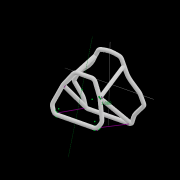
# Autodesk Inventor part: profiles
Saved by Autodesk Inventor 2020 (Build 240168000, 168)
## iProperties
Created: 2020-03-12
Part Number: profiles
Material: Generic
Document SubType Name: Modeling
Designer: valer
Density: 1 g/cm^3
Appearance: Default
Author: valer
Autodesk Inventor part; units mm, degrees
ref_plane "YZ Plane" through (0, 0, 0) normal (1, 0, 0) x (0, 1, 0)
ref_plane "XZ Plane" through (0, 0, 0) normal (0, 1, 0) x (-1, 0, 0)
sketch "FrontTube" plane through (0, 0, 0) normal (1, 0, 0) x (0, 1, 0)
  circle A0 centre (203.2, 0) radius 12.7
  line L0 (-302.2779, 0) -> (302.263, 0) projected
  point P0 (0, 0)
  dimension "d35" = 25.4
  constraints: 1 centre point, 1 point on line
  measures "d35" diameter of A0
sketch "Front1" plane through (0, 0, 0) normal (0, 0, 1) x (1, 0, 0)
  arc A0 (63.0606, 202.3316) -> (0.9117, 211.6354) centre (-9.1171, -67.5845) ccw
  arc A1 (86.36, 182.4422) -> (63.0606, 202.3316) centre (53.8743, 167.9787) ccw
  line L0 (0, 211.6667) -> (0, -211.6667) construction
  line L1 (86.36, 182.4422) -> (117.3533, 112.8301)
  line L2 (149.1123, 68.3056) -> (198.6494, 22.1116)
  line L3 (213.8608, 1.1748) -> (235.3298, -44.8656)
  line L4 (232.2048, -71.3906) -> (184.8333, -131.0763)
  line L5 (137.16, -211.6667) -> (0, -211.6667)
  line L6 (170.9584, -158.5658) -> (161.6802, -192.894)
  arc A2 (117.3533, 112.8301) -> (149.1123, 68.3056) centre (242.6552, 168.6181) ccw
  arc A3 (137.16, -211.6667) -> (161.6802, -192.894) centre (137.16, -186.2667) ccw
  arc A4 (184.8333, -131.0763) -> (170.9584, -158.5658) centre (244.5189, -178.4478) ccw
  arc A5 (232.2048, -71.3906) -> (235.3298, -44.8656) centre (212.3096, -55.6001) ccw
  arc A6 (213.8608, 1.1748) -> (198.6494, 22.1116) centre (152.4, -27.4848) ccw
  arc A7 (-0.9117, 211.6354) -> (-63.0606, 202.3316) centre (9.1171, -67.5845) ccw
  arc A8 (-63.0606, 202.3316) -> (-86.36, 182.4422) centre (-53.8743, 167.9787) ccw
  line L7 (-86.36, 182.4422) -> (-117.3533, 112.8301)
  line L8 (-149.1123, 68.3056) -> (-198.6494, 22.1116)
  line L9 (-213.8608, 1.1748) -> (-235.3298, -44.8656)
  line L10 (-232.2048, -71.3906) -> (-184.8333, -131.0763)
  line L11 (-137.16, -211.6667) -> (0, -211.6667)
  line L12 (-170.9584, -158.5658) -> (-161.6802, -192.894)
  arc A9 (-149.1123, 68.3056) -> (-117.3533, 112.8301) centre (-242.6552, 168.6181) ccw
  arc A10 (-161.6802, -192.894) -> (-137.16, -211.6667) centre (-137.16, -186.2667) ccw
  arc A11 (-170.9584, -158.5658) -> (-184.8333, -131.0763) centre (-244.5189, -178.4478) ccw
  arc A12 (-235.3298, -44.8656) -> (-232.2048, -71.3906) centre (-212.3096, -55.6001) ccw
  arc A13 (-198.6494, 22.1116) -> (-213.8608, 1.1748) centre (-152.4, -27.4848) ccw
  arc A14 (0.9117, 211.6354) -> (-0.9117, 211.6354) centre (0, 186.2518) ccw
  point P0 (0, 0)
  point P1 (0, 0)
  dimension "d15" = 86.36
  dimension "d16" = 25.4
  dimension "d17" = 25.4
  dimension "d18" = 76.2
  dimension "d19" = 25
  dimension "d20" = 47
  dimension "d21" = 24
  dimension "d22" = 137.16
  dimension "d23" = 279.4
  dimension "d24" = 35.56
  dimension "d25" = 76.2
  dimension "d26" = 137.16
  dimension "d27" = 67.7333
  dimension "d28" = 50.8
  dimension "d29" = 76.2
  dimension "d30" = 35.56
  dimension "d32" = 152.4
  dimension "d33" = 43.688
  dimension "d34" = 423.3333
  dimension "d38" = 25.4
  constraints: 32 point on circle, 26 end point, 19 symmetric about line, 15 centre point, 14 tangent, 1 midpoint, 1 perpendicular, 1 vertical, 7 other
  measures "d15" distance from line of L1.start L0
  measures "d16" radius of A3
  measures "d17" radius of A5
  measures "d18" radius of A4
  measures "d19" angle of L0 L3
  measures "d20" angle of L0 L2
  measures "d21" angle of L0 L1
  measures "d22" distance of L5.start L0.end
  measures "d23" radius of A0
  measures "d24" radius of A1
  measures "d25" distance of L1.start L1.end
  measures "d26" radius of A2
  measures "d27" distance of L2.start L2.end
  measures "d28" distance of L3.start L3.end
  measures "d29" distance of L4.start L4.end
  measures "d30" distance of L6.start L6.end
  measures "d32" distance from line of L0 A6.centre
  measures "d33" vertical distance of A1.centre L0.start
  measures "d34" distance of L0.end L0.start
  measures "d38" radius of A14
sweep "Front1Feature" add profiles "FrontTube" path "Front1" path curves A0 A1 L1 A2 L2 A6 L3 A5 L4 A4 L6 A3 L5 L11 A10 L12 A11 L10 A12 L9 A13 L8 A9 L7 A8 A7 A14
ref_plane "MiddlePlane" through (0, 0, 254) normal (0, 0, 1) x (1, 0, 0)
sketch "MiddleEdge" plane through (0, 0, 254) normal (0, 0, 1) x (1, 0, 0)
  line L0 (-31.1191, 127.0482) -> (68.8934, 127.0482)
  point P0 (0, 0)
  constraints: 2 end point, 1 horizontal
ref_plane "MiddleRotatedPlane" through (-31.1191, 127.0482, 254) normal (0, 0.309017, 0.9510565) x (1, 0, 0)
ref_plane "BackPlane" through (0, 0, 457.2) normal (0, 0, 1) x (1, 0, 0)
sketch "Middle" plane through (-31.1191, 127.0482, 254) normal (0, 0.309017, 0.9510565) x (1, 0, 0)
  line L0 (31.1191, 38.7554) -> (75.1914, 38.7554)
  line L1 (105.257, 22.1842) -> (149.4691, -47.8183)
  line L2 (180.8254, -206.284) -> (188.7793, -192.1968)
  line L3 (154.4333, -58.0694) -> (191.3548, -162.9001)
  line L4 (31.1191, -224.3603) -> (149.8603, -224.3603)
  line L5 (31.1191, 38.7554) -> (31.1191, -224.3603) construction
  arc A0 (105.257, 22.1842) -> (75.1914, 38.7554) centre (75.1914, 3.1954) ccw
  arc A1 (154.4333, -58.0694) -> (149.4691, -47.8183) centre (106.5183, -74.9451) ccw
  arc A2 (188.7793, -192.1968) -> (191.3548, -162.9001) centre (157.8143, -174.7131) ccw
  arc A3 (149.8603, -224.3603) -> (180.8254, -206.284) centre (149.8603, -188.8003) ccw
  line L6 (31.1191, 38.7554) -> (-12.9532, 38.7554)
  line L7 (-43.0188, 22.1842) -> (-87.2309, -47.8183)
  line L8 (-118.5871, -206.284) -> (-126.5411, -192.1968)
  line L9 (-92.1951, -58.0694) -> (-129.1166, -162.9001)
  line L10 (31.1191, -224.3603) -> (-87.6221, -224.3603)
  arc A4 (-12.9532, 38.7554) -> (-43.0188, 22.1842) centre (-12.9532, 3.1954) ccw
  arc A5 (-87.2309, -47.8183) -> (-92.1951, -58.0694) centre (-44.2801, -74.9451) ccw
  arc A6 (-129.1166, -162.9001) -> (-126.5411, -192.1968) centre (-95.5761, -174.7131) ccw
  arc A7 (-118.5871, -206.284) -> (-87.6221, -224.3603) centre (-87.6221, -188.8003) ccw
  line L11 (31.1191, 38.7554) -> (31.1191, 45.1054) construction
  line L12 (31.1191, -224.3603) -> (31.1191, -275.1603) construction
  point P0 (31.1191, -42.3397)
  dimension "d86" = 35.56
  dimension "d87" = 50.8
  dimension "d88" = 35.56
  dimension "d98" = 50.8
  constraints: 26 end point, 16 point on circle, 12 symmetric about line, 8 centre point, 8 tangent, 3 vertical, 2 horizontal, 1 equal radius, 4 other
  measures "d86" radius of A0
  measures "d87" radius of A1
  measures "d88" radius of A2
  measures "d98" distance of L4.start L12.end
sketch "MiddleTube" plane through (0, 0, 0) normal (1, 0, 0) x (0, 1, 0)
  circle A0 centre (163.9068, 242.0239) radius 12.7
  point P0 (0, 0)
  dimension "d89" = 25.4
  constraints: 1 centre point, 1 coincident
  measures "d89" diameter of A0
sweep "MiddleFeature" add profiles "MiddleTube" path "Middle" separate body path curves L6 A4 L7 A5 L9 A6 L8 A7 L10 L4 A3 L2 A2 L3 A1 L1 A0 L0
sketch "BackProfile" plane through (0, 0, 457.2) normal (0, 0, 1) x (1, 0, 0)
  line L0 (41.4631, 93.1618) -> (47.5828, 84.9091)
  line L1 (0, 100.0125) -> (27.8545, 100.0125)
  line L2 (50.6768, 77.6546) -> (60.2398, 21.3464)
  line L3 (0, 1.5679) -> (43.5372, 1.5679)
  line L4 (0, 100.0125) -> (0, 1.5679) construction
  arc A0 (41.4631, 93.1618) -> (27.8545, 100.0125) centre (27.8545, 83.0707) ccw
  arc A1 (50.6768, 77.6546) -> (47.5828, 84.9091) centre (33.9742, 74.8179) ccw
  arc A2 (43.5372, 1.5679) -> (60.2398, 21.3464) centre (43.5372, 18.5097) ccw
  line L5 (-41.4631, 93.1618) -> (-47.5828, 84.9091)
  line L6 (0, 100.0125) -> (-27.8545, 100.0125)
  line L7 (-50.6768, 77.6546) -> (-60.2398, 21.3464)
  line L8 (0, 1.5679) -> (-43.5372, 1.5679)
  arc A3 (-27.8545, 100.0125) -> (-41.4631, 93.1618) centre (-27.8545, 83.0707) ccw
  arc A4 (-47.5828, 84.9091) -> (-50.6768, 77.6546) centre (-33.9742, 74.8179) ccw
  arc A5 (-60.2398, 21.3464) -> (-43.5372, 1.5679) centre (-43.5372, 18.5097) ccw
  line L9 (0, 100.0125) -> (0, 125.3956) construction
  point P0 (0, 0)
  dimension "d92" = 16.9418
  dimension "d93" = 16.9418
  dimension "d97" = 25.3831
  constraints: 20 end point, 12 point on circle, 9 symmetric about line, 6 centre point, 6 tangent, 2 horizontal, 2 vertical, 1 equal radius, 3 other
  measures "d92" radius of A0
  measures "d93" radius of A2
  measures "d97" distance of L1.start L9.end
sketch "BackTube" plane through (0, 0, 0) normal (1, 0, 0) x (0, 1, 0)
  circle A0 centre (100.0125, 457.2) radius 12.7
  point P0 (0, 0)
  point P1 (100.0125, 457.2)
  point P2 (100.0125, 457.2)
  point P3 (100.0125, 457.2)
  dimension "d94" = 25.4
  constraints: 1 centre point, 1 coincident
  measures "d94" diameter of A0
feature "BackFeature" [suppressed]
sketch "FrontTopTubes" plane through (0, 0, 0) normal (0, 0, 1) x (1, 0, 0)
  circle A0 centre (94.1356, 144.1985) radius 12.7
  line L0 (57.5964, 181.8978) -> (64.158, 206.4357) projected
  line L1 (0.6083, 203.1891) -> (0.6083, 203.1891) projected
  line L2 (0.6083, 203.1891) -> (0.6083, 203.1891) projected
  line L3 (-0.1525, 190.4973) -> (-1.0642, 215.8809) projected
  line L4 (-57.5964, 181.8978) -> (-64.158, 206.4357) projected
  line L5 (-137.16, -190.5149) -> (-137.16, -215.9149) projected
  line L6 (137.16, -190.5149) -> (137.16, -215.9149) projected
  line L7 (98.0302, 104.2269) -> (121.2343, 114.558) construction
  line L8 (67.0369, 173.839) -> (90.2409, 184.1701) projected
  line L9 (90.2409, 184.1701) -> (121.2343, 114.558) construction
  line L10 (67.0369, 173.839) -> (98.0302, 104.2269) construction
  line L11 (67.0369, 173.839) -> (90.2409, 184.1701) projected
  line L12 (0, -302.274) -> (0, 302.2401) construction
  circle A1 centre (-94.1356, 144.1985) radius 12.7
  circle A2 centre (147.4628, -199.7238) radius 12.7
  circle A3 centre (-147.4628, -199.7238) radius 12.7
  arc A4 (-141.2611, -187.3751) -> (-137.16, -190.5149) centre (-137.16, -186.2667) ccw projected
  arc A5 (-165.7812, -194.0025) -> (-137.16, -215.9149) centre (-137.16, -186.2667) ccw projected
  arc A6 (137.16, -215.9149) -> (165.7812, -194.0025) centre (137.16, -186.2667) ccw projected
  point P0 (0, 0)
  point P1 (155.1831, -209.8078)
  point P2 (-155.1831, -209.8078)
  dimension "d99" = 25.4
  dimension "d100" = 38.1
  constraints: 2 centre point, 2 coincident, 2 point on circle, 1 symmetric about line, 1 tangent, 10 other
  measures "d99" diameter of A0
  measures "d100" distance from line of L8 A0.centre
sketch "MiddleTopTubes" plane through (-31.1191, 127.0482, 254) normal (0, 0.309017, 0.9510565) x (1, 0, 0)
  circle A0 centre (152.2394, -52.8043) radius 12.7
  line L0 (115.9947, 28.9659) -> (94.5193, 15.4025) construction
  line L1 (31.1191, -430.2644) -> (31.1191, 261.8485) construction
  circle A1 centre (-90.0012, -52.8043) radius 12.7
  arc A2 (142.4545, -62.2883) -> (138.7314, -54.6) centre (106.5183, -74.9451) ccw projected
  arc A3 (166.4121, -53.8505) -> (160.2068, -41.0366) centre (106.5183, -74.9451) ccw projected
  circle A4 centre (167.7879, -219.5105) radius 12.7
  circle A5 centre (-105.5496, -219.5105) radius 12.7
  arc A6 (149.8603, -237.0603) -> (191.8843, -212.5281) centre (149.8603, -188.8003) ccw projected
  arc A7 (149.8603, -211.6603) -> (169.7664, -200.0398) centre (149.8603, -188.8003) ccw projected
  arc A8 (-129.6461, -212.5281) -> (-87.6221, -237.0603) centre (-87.6221, -188.8003) ccw projected
  arc A9 (-107.5282, -200.0398) -> (-87.6221, -211.6603) centre (-87.6221, -188.8003) ccw projected
  point P0 (31.1191, -42.3397)
  point P1 (163.6697, -47.269)
  point P2 (174.1906, -230.4784)
  point P3 (-111.9523, -230.4784)
  dimension "d106" = 25.4
  constraints: 3 point on circle, 2 coincident, 1 centre point, 1 symmetric about line, 13 other
sketch3d "TopTubeLeft"
  line L0 (121.1203, 76.8284, 270.3174) -> (94.1356, 144.1985, 0)
sweep "TopTubeLeftFeature" add profiles "MiddleTopTubes" path "TopTubeLeft" separate body contours A0
sketch3d "TopTubeRight"
  line L0 (-94.1356, 144.1985, 0) -> (-121.1203, 76.8284, 270.3174)
sweep "TopTubeRightFeature" add profiles "FrontTopTubes" path "TopTubeRight" separate body contours A1
sketch3d "BottomTubeRight"
sketch3d "BottomTubeLeft"
ref_plane "SideTubeRightPlane" through (121.1203, 76.8284, 270.3174) normal (0.0679602, -0.7134686, -0.6973837) x (0.995494, 0.0948241, 0)
ref_plane "SideTubeLeftPlane" through (-121.1203, 76.8284, 270.3174) normal (0.0679602, 0.7134686, 0.6973837) x (-0.995494, 0.0948241, 0)
sketch "SideTubeRightProfile" plane through (121.1203, 76.8284, 270.3174) normal (0.0679602, -0.7134686, -0.6973837) x (0.995494, 0.0948241, 0)
  circle A0 centre (0, 0) radius 12.7
  ellipse E0 centre (0, 0) end of major axis (12.6751, -0.7952) minor radius 11.2233 projected
  point P0 (-127.8597, -148.408)
  dimension "d113" = 25.4
  constraints: 1 centre point, 1 coincident
  measures "d113" diameter of A0
sketch "SideTubeLeftProfile" plane through (-121.1203, 76.8284, 270.3174) normal (0.0679602, 0.7134686, 0.6973837) x (-0.995494, 0.0948241, 0)
  ellipse E0 centre (0, 0) end of major axis (-12.6751, 0.7952) minor radius 11.2233 projected
  circle A0 centre (0, 0) radius 12.7
  point P0 (-127.8597, -148.408)
  dimension "d114" = 25.4
  constraints: 1 centre point, 1 coincident, 1 other
  measures "d114" diameter of A0
sketch3d "SideTubeRight"
  line L0 (121.1203, 76.8284, 270.3174) -> (147.4628, -199.7238, 0)
sweep "SideTubeRightFeature" add profiles "SideTubeRightProfile" path "SideTubeRight" separate body
sketch3d "SideTubeLeft"
  line L0 (-121.1203, 76.8284, 270.3174) -> (-147.4628, -199.7238, 0)
sweep "SideTubeLeftFeature" add profiles "SideTubeLeftProfile" path "SideTubeLeft" separate body
ref_plane "BottomTubeRightPlane" through (136.6687, -81.7187, 321.8325) normal (0.0314737, -0.3440838, -0.9384113) x (0.9958426, 0.0910907, 0)
ref_plane "BottomTubeLeftPlane" through (-136.6687, -81.7187, 321.8325) normal (-0.0314737, -0.3440838, -0.9384113) x (0.9958426, -0.0910907, 0)
body "Solid1"
body "Solid5"
body "Solid6"
body "Solid7"
body "Solid8"
body "Solid13"
body "Solid14"
